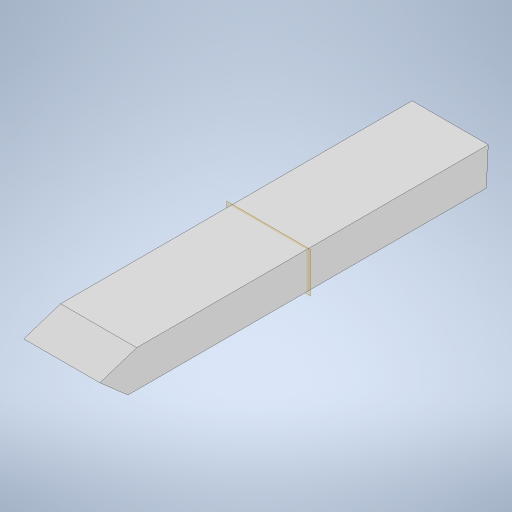
# Autodesk Inventor part: Enemy_hull_collision
Saved by Autodesk Inventor 2024 (Build 280153000, 153)
## iProperties
Created: 2026-05-20
Part Number: Enemy_hull_collision
Material: Generic
Document SubType Name: Modeling
Designer: warny
Density: 1 g/cm^3
Appearance: Default
Author: warny
Autodesk Inventor part; units mm, degrees
ref_plane "YZ Plane" through (0, 0, 0) normal (1, 0, 0) x (0, 1, 0)
ref_plane "XZ Plane" through (0, 0, 0) normal (0, 1, 0) x (-1, 0, 0)
sketch "Sketch2" plane through (0, 0, 0) normal (1, 0, 0) x (0, 1, 0)
  line L0 (0, -524.16) -> (0, 575.96) projected
  line L1 (0, 361.9) -> (49.78, 418.8)
  line L2 (49.78, 418.8) -> (74.08, 344.3)
  line L3 (74.08, 344.3) -> (74.08, -367)
  line L4 (74.08, -367) -> (0, -363)
  line L5 (0, -363) -> (0, 0)
  line L6 (0, 361.9) -> (0, 0)
  dimension "d0" = 361.9
  dimension "d1" = 56.9
  dimension "d2" = 49.78
  dimension "d3" = 24.3
  dimension "d4" = 74.5
  dimension "d5" = 363
  dimension "d6" = 4
  dimension "d7" = 74.08
  constraints: 12 end point, 2 collinear, 2 point on line
  measures "d0" distance of L5.end L1.start
  measures "d1" vertical distance of L1.start L1.end
  measures "d2" horizontal distance of L1.end L1.start
  measures "d3" horizontal distance of L1.end L2.end
  measures "d4" vertical distance of L2.end L1.end
  measures "d5" distance of L5.end L4.end
  measures "d6" vertical distance of L3.end L4.end
  measures "d7" horizontal distance of L3.end L4.end
extrude "Extrusion1" add sketch "Sketch2" along normal mid plane 154
body "Solid1"
